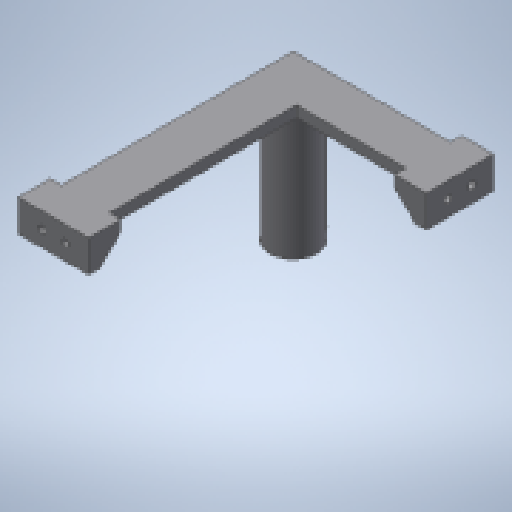
# Autodesk Inventor part: SpoolHolder
Saved by Autodesk Inventor 2023 (Build 270158000, 158)
## iProperties
Created: 2022-09-12
Part Number: SpoolHolder
Material: PET Plastic
Document SubType Name: Modeling
Designer: Nathann
Density: 1.541 g/cm^3
Appearance: Polycarbonate - Clear
Author: Nathann
Autodesk Inventor part; units mm, degrees
ref_plane "YZ Plane" through (0, 0, 0) normal (1, 0, 0) x (0, 1, 0)
ref_plane "XZ Plane" through (0, 0, 0) normal (0, 1, 0) x (-1, 0, 0)
ref_plane "XY Plane" through (0, 0, 0) normal (0, 0, 1) x (1, 0, 0)
sketch "Sketch1" plane through (0, 0, 0) normal (1, 0, 0) x (0, 1, 0)
  line L0 (0, 0) -> (-20, 0)
  line L1 (-20, 0) -> (-20, -7)
  line L2 (-20, -7) -> (0, -7)
  line L3 (0, -7) -> (0, 0)
  line L4 (0, -7) -> (-7, -7)
  line L5 (-7, -7) -> (-7, -150)
  line L6 (-7, -150) -> (0, -150)
  line L7 (0, -150) -> (0, -7)
  dimension "d0" = 7
  dimension "d1" = 20
  dimension "d2" = 7
  dimension "d3" = 150
  constraints: 16 end point, 4 parallel, 2 horizontal, 2 perpendicular
  measures "d0" distance of L0.end L1.end
  measures "d1" distance of L0.start L0.end
  measures "d2" distance between parallel lines of L5 L7
  measures "d3" distance between parallel lines of L6 L0
extrude "Extrusion1" add sketch "Sketch1" along normal blind 30
sketch "Sketch2" plane through (0, -7, -150) normal (0, -1, 0) x (1, 0, 0)
  line L0 (0, 0) -> (30, 0) projected
  circle A0 centre (15, 0) radius 15
  point P0 (0, 150)
  constraints: 1 horizontal alignment, 1 midpoint, 2 other
extrude "Extrusion2" add sketch "Sketch2" along normal blind 80 and the other way blind 7
sketch "Sketch3" plane through (0, -20, -7) normal (0, 0, -1) x (-1, 0, 0)
  circle A0 centre (-7.5, 10) radius 2.25
  circle A1 centre (-22.5, 10) radius 2.25
  line L0 (0, 0) -> (-30, 0) projected
  line L1 (-30, 0) -> (-30, 13) projected
  point P0 (0, 20)
  dimension "d10" = 10
  dimension "d11" = 4.5
  dimension "d12" = 4.5
  dimension "d13" = 10
  dimension "d14" = 15
  dimension "d15" = 7.5
  constraints: 2 centre point
  measures "d10" distance from line of A0.centre L0
  measures "d11" diameter of A0
  measures "d12" diameter of A1
  measures "d13" distance from line of L0 A1.centre
  measures "d14" distance of A1.centre A0.centre
  measures "d15" distance from line of L1 A1.centre
sketch "Sketch4" plane through (30, 0, 0) normal (1, 0, 0) x (0, 0, -1)
  line L0 (150, 0) -> (0, 0) projected
  line L1 (0, 0) -> (0, -20) projected
  line L2 (0, -20) -> (7, -20) projected
  line L3 (7, -20) -> (7, -7) projected
  line L4 (7, -7) -> (150, -7) projected
  line L5 (150, -7) -> (150, 0) projected
  line L6 (7, -20) -> (7, -7) projected
  line L7 (7, -20) -> (20, -7)
  line L8 (7, -7) -> (150, -7) projected
  line L9 (20, -7) -> (20, 0)
  dimension "d16" = 13
  constraints: 4 end point, 2 point on line, 1 perpendicular
  measures "d16" distance between parallel lines of L3 L9
extrude "Extrusion3" add sketch "Sketch4" along normal blind 7 contours L9 L4 L3 L2 L1 L0 | L7 L3 L4
extrude "Extrusion4" cut sketch "Sketch3" against normal blind 7
sketch "Sketch5" plane through (0, 0, 0) normal (-1, 0, 0) x (0, 0, 1)
  line L0 (-150, 0) -> (0, 0) projected
  line L1 (-150, -7) -> (-150, 0) projected
  line L2 (-7, -7) -> (-150, -7) projected
  line L3 (-7, -20) -> (-7, -7) projected
  line L4 (0, -20) -> (-7, -20) projected
  line L5 (0, 0) -> (0, -20) projected
  line L6 (-7, -20) -> (-20, -7) projected
  line L7 (-7, -20) -> (-20, -7)
  line L8 (-20, 0) -> (-20, -7) projected
  line L9 (-20, -7) -> (-20, 0)
  constraints: 4 end point, 2 collinear
extrude "Extrusion5" add sketch "Sketch5" along normal blind 7 contours L0 L5 L4 L3 L2 L8 | L2 L3 L6
sketch "Sketch6" plane through (30, -20, -7) normal (0, 0, -1) x (-1, 0, 0)
  circle A0 centre (7.5, 10) radius 2.25 projected
  circle A1 centre (22.5, 10) radius 2.25 projected
  circle A2 centre (7.5, 10) radius 5.5
  circle A3 centre (22.5, 10) radius 5.5
  point P0 (30, 20)
  dimension "d23" = 11
  dimension "d24" = 11
  constraints: 2 centre point, 2 coincident
  measures "d23" diameter of A2
  measures "d24" diameter of A3
extrude "Extrusion6" cut sketch "Sketch6" along normal blind 12
sketch "Sketch7" plane through (0, 0, 0) normal (-1, 0, 0) x (0, 0, 1)
  line L0 (-193.0937, 8.1233) -> (-158, 8.1233)
  line L1 (-158, 8.1233) -> (-158, -80)
  line L2 (-158, -80) -> (-193.0937, -80)
  line L3 (-193.0937, -80) -> (-193.0937, 8.1233)
  line L4 (-150, 0) -> (-165, 0) projected
  point P0 (0, 0)
  dimension "d27" = 80
  dimension "d28" = 7
  constraints: 8 end point, 2 parallel, 1 horizontal, 1 perpendicular
  measures "d27" distance between parallel lines of L2 L4
  measures "d28" distance from line of L4.end L1
extrude "Extrusion7" cut sketch "Sketch7" against normal blind 72
sketch "Sketch8" plane through (30, 0, -20) normal (0, 1, 0) x (1, 0, 0)
  line L0 (0, 145) -> (-118.3328, 145)
  line L1 (-118.3328, 145) -> (-118.3328, 116.9928)
  line L2 (-118.3328, 116.9928) -> (0, 116.9928)
  line L3 (0, 116.9928) -> (0, 145)
  line L4 (0, 130) -> (0, 0) projected
  arc A0 (-2.3114, 138) -> (-27.6886, 138) centre (-15, 130) ccw projected
  line L5 (-138.3328, 520) -> (-138.3328, -40) projected
  point P0 (-30, -20)
  dimension "d31" = 0
  dimension "d32" = 15
  dimension "d33" = 20
  constraints: 8 end point, 2 parallel, 1 horizontal, 1 perpendicular
  measures "d31" distance between parallel lines of L4 L3
  measures "d32" distance from line of A0.centre L0
  measures "d33" distance between parallel lines of L1 L5
extrude "Extrusion8" add sketch "Sketch8" against normal blind 7
sketch "Sketch9" plane through (30, -7, -150) normal (0, -1, 0) x (1, 0, 0)
  line L0 (-118.3328, -22) -> (-111.3328, -22)
  line L1 (-111.3328, -22) -> (-111.3328, 20.0072)
  line L2 (-111.3328, 20.0072) -> (-118.3328, 20.0072)
  line L3 (-118.3328, 20.0072) -> (-118.3328, -22)
  line L4 (-118.3328, 13.0072) -> (-118.3328, -15) projected
  line L5 (-30, 13.0072) -> (-118.3328, 13.0072) projected
  line L6 (-118.3328, -15) -> (0, -15) projected
  point P0 (-30, 150)
  dimension "d36" = 7
  dimension "d37" = 0
  dimension "d38" = 7
  dimension "d39" = 7
  constraints: 8 end point, 2 parallel, 1 horizontal, 1 perpendicular
  measures "d36" distance between parallel lines of L3 L1
  measures "d37" distance between parallel lines of L4 L3
  measures "d38" distance between parallel lines of L5 L2
  measures "d39" distance between parallel lines of L0 L6
extrude "Extrusion9" add sketch "Sketch9" along normal blind 13 and the other way blind 7
sketch "Sketch10" plane through (-81.3328, -20, -172) normal (0, 0, -1) x (-1, 0, 0)
  line L0 (7, 0) -> (0, 0) projected
  line L1 (0, 0) -> (-20, 20)
  line L2 (0, 20) -> (-81.3328, 20) projected
  line L3 (0, 20) -> (0, 0) projected
  line L4 (0, 13) -> (-111.3328, 13) projected
  line L5 (-13, 13) -> (-13, 20)
  dimension "d44" = 45
  constraints: 4 end point, 4 point on line, 1 perpendicular
  measures "d44" angle of L3 L1
extrude "Extrusion10" add sketch "Sketch10" against normal blind 7 contours L1 L4 L3 | L5 L2 L3 L4
sketch "Sketch11" plane through (-88.3328, -20, -129.9928) normal (0, 0, 1) x (1, 0, 0)
  line L0 (7, 0) -> (7, 13) projected
  line L1 (20, 13) -> (27, 20) projected
  line L2 (7, 0) -> (20, 13)
  line L3 (20, 13) -> (20, 20)
  line L4 (0, 20) -> (20, 20) projected
  line L5 (7, 20) -> (7, 13)
  line L6 (7, 20) -> (7, 13) projected
  line L7 (7, 20) -> (20, 20)
  point P0 (88.3328, 20)
  constraints: 9 end point, 1 collinear, 1 parallel, 1 perpendicular, 1 point on line, 1 vertical
extrude "Extrusion11" add sketch "Sketch11" against normal blind 7
sketch "Sketch13" plane through (-81.3328, -20, -165) normal (1, 0, 0) x (0, 0, -1)
  circle A0 centre (-6.5, 10) radius 2.25
  circle A1 centre (-21.5, 10) radius 2.25
  line L0 (0, 0) -> (-28.0072, 0) projected
  line L1 (-158, 12.25) -> (-158, 7.75) projected
  line L2 (-158, 12.25) -> (-158, 7.75) projected
  line L3 (0, 0) -> (0, 13) projected
  line L4 (-28.0072, 13) -> (-28.0072, 0) projected
  point P0 (-165, 20)
  dimension "d49" = 10
  dimension "d50" = 10
  dimension "d51" = 15
  dimension "d52" = 6.5
  dimension "d53" = 6.5072
  dimension "d54" = 4.5
  dimension "d55" = 4.5
  constraints: 2 centre point
  measures "d49" distance from line of L0 A0.centre
  measures "d50" distance from line of L0 A1.centre
  measures "d51" distance of A1.centre A0.centre
  measures "d52" distance from line of L3 A0.centre
  measures "d53" distance from line of A1.centre L4
  measures "d54" diameter of A0
  measures "d55" diameter of A1
extrude "Extrusion12" cut sketch "Sketch13" against normal blind 7
sketch "Sketch15" plane through (-81.3328, -20, -165) normal (1, 0, 0) x (0, 0, -1)
  circle A0 centre (-6.5, 10) radius 2.25 projected
  circle A1 centre (-6.5, 10) radius 5
  circle A2 centre (-21.5, 10) radius 2.25 projected
  circle A3 centre (-21.5, 10) radius 5
  point P0 (-165, 20)
  dimension "d58" = 10
  dimension "d59" = 10
  constraints: 2 centre point, 2 coincident
  measures "d58" diameter of A1
  measures "d59" diameter of A3
extrude "Extrusion13" cut sketch "Sketch15" along normal blind 20 contours A1 | A2 | A3
mirror "Mirror1" about plane through (37, -10, -10) normal (1, 0, 0) of "Extrusion13", "Extrusion12", "Extrusion11", "Extrusion10", "Extrusion9", "Extrusion8", "Extrusion7", "Extrusion6", "Extrusion5", "Extrusion4", "Extrusion3", "Extrusion2", "Extrusion1"
sketch "Sketch16" plane through (27.6886, -80, -158) normal (0, 0, -1) x (-1, 0, 0)
  line L0 (34.6886, 80) -> (-53.3114, 80) projected
  line L1 (-9.3114, 80) -> (-9.3114, -30.4412)
  line L2 (-9.3114, -30.4412) -> (154.0153, -30.4412)
  line L3 (154.0153, -30.4412) -> (154.0153, 105.4086)
  line L4 (154.0153, 105.4086) -> (-9.3114, 105.4086)
  line L5 (-9.3114, 105.4086) -> (-9.3114, -30.4412)
  point P0 (27.6886, 80)
  constraints: 10 end point, 2 parallel, 1 horizontal, 1 midpoint, 1 perpendicular, 1 vertical
extrude "Extrusion14" cut sketch "Sketch16" along normal mid plane 400
equation "\"d12\" = d11"
equation "\"d13\" = d10"
body "Solid1"
